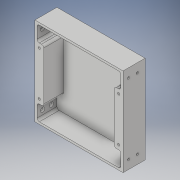
# Autodesk Inventor part: wheel core
Saved by Autodesk Inventor 2018 (Build 220112000, 112)
## iProperties
Created: 2018-08-07
Part Number: wheel core
Material: Generic
Document SubType Name: Modeling
Designer: Cole Tucker
Density: 1 g/cm^3
Appearance: Default
Author: Cole Tucker
Autodesk Inventor part; units mm, degrees
ref_plane "YZ Plane" through (0, 0, 0) normal (1, 0, 0) x (0, 1, 0)
ref_plane "XZ Plane" through (0, 0, 0) normal (0, 1, 0) x (-1, 0, 0)
sketch "Sketch1" plane through (0, 0, 0) normal (0, 0, 1) x (1, 0, 0)
  line L0 (0, 0) -> (127, 0)
  line L1 (127, 0) -> (127, 127)
  line L2 (127, 127) -> (0, 127)
  line L3 (0, 127) -> (0, 0)
  dimension "d0" = 127
  dimension "d1" = 127
  constraints: 8 end point, 2 parallel, 1 horizontal, 1 perpendicular
  measures "d0" distance of L2.end L1.end
  measures "d1" distance of L1.end L0.end
extrude "Extrusion1" add sketch "Sketch1" along normal blind 31.75
shell "Shell1" thickness 3.175 removed faces 1 at (42.3333, 84.6667, 31.75)
sketch "Sketch3" plane through (3.175, 3.175, 3.175) normal (1, 0, 0) x (0, 0, -1)
  line L0 (0, 0) -> (-28.575, 0) construction
  line L1 (-14.2875, 0) -> (-14.2875, 120.65) construction
  line L2 (0, 120.65) -> (-28.575, 120.65) construction
  line L3 (-14.2875, 120.65) -> (-20.6375, 120.65) construction
  line L4 (-20.6375, 120.65) -> (-20.6375, 111.125) construction
  line L5 (-20.6375, 111.125) -> (-14.2875, 111.125) construction
  line L6 (-14.2875, 111.125) -> (-14.2875, 120.65) construction
  line L7 (-14.2875, 120.65) -> (-7.9375, 120.65) construction
  line L8 (-7.9375, 120.65) -> (-7.9375, 111.125) construction
  line L9 (-7.9375, 111.125) -> (-14.2875, 111.125) construction
  line L10 (-14.2875, 111.125) -> (-14.2875, 120.65) construction
  line L11 (-14.2875, 0) -> (-20.6375, 0) construction
  line L12 (-20.6375, 0) -> (-20.6375, 9.525) construction
  line L13 (-20.6375, 9.525) -> (-14.2875, 9.525) construction
  line L14 (-14.2875, 9.525) -> (-14.2875, 0) construction
  line L15 (-14.2875, 0) -> (-7.9375, 0) construction
  line L16 (-7.9375, 0) -> (-7.9375, 9.525) construction
  line L17 (-7.9375, 9.525) -> (-14.2875, 9.525) construction
  line L18 (-14.2875, 9.525) -> (-14.2875, 0) construction
  point P0 (3.175, -3.175)
  dimension "d5" = 6.35
  dimension "d6" = 9.525
  dimension "d7" = 6.35
  dimension "d8" = 6.35
  dimension "d9" = 9.525
  dimension "d10" = 6.35
  dimension "d11" = 9.525
  constraints: 34 end point, 8 parallel, 4 coincident, 4 horizontal, 4 perpendicular, 2 midpoint, 1 point on line
  measures "d5" distance of L5.end L4.end
  measures "d6" distance of L4.end L3.end
  measures "d7" distance of L8.end L9.end
  measures "d8" distance of L12.end L13.end
  measures "d9" distance of L11.end L12.end
  measures "d10" distance of L17.end L16.end
  measures "d11" distance of L16.end L15.end
hole "Hole1" at (3.175, 12.7, 23.8125) at (3.175, 12.7, 11.1125) at (3.175, 114.3, 23.8125) at (3.175, 114.3, 11.1125) direction (-1, 0, 0) diameter 3.175 depth 15.6718 tip angle 118 countersink diameter 6.35 countersink angle 82
ref_plane "Work Plane1" through (63.5, 0, 0) normal (1, 0, 0) x (0, 0, -1)
sketch "Sketch4" plane through (3.175, 3.175, 3.175) normal (0, 0, 1) x (1, 0, 0)
  line L0 (0, 0) -> (0, 120.65) construction
  line L1 (0, 120.65) -> (0, 98.425) construction
  line L2 (0, 0) -> (120.65, 0) construction
  line L3 (0, 0) -> (0, 22.225) construction
  line L4 (0, 98.425) -> (9.525, 98.425)
  line L5 (9.525, 98.425) -> (9.525, 22.225)
  line L6 (9.525, 22.225) -> (0, 22.225)
  line L7 (0, 22.225) -> (0, 98.425)
  point P0 (-3.175, -3.175)
  dimension "d19" = 22.225
  dimension "d20" = 22.225
  dimension "d21" = 9.525
  constraints: 12 end point, 2 parallel, 2 point on line, 1 horizontal, 1 perpendicular
  measures "d19" distance of L0.end L1.end
  measures "d20" distance of L0.start L3.end
  measures "d21" distance of L5.end L6.end
extrude "Extrusion2" add sketch "Sketch4" along normal up to surface (28.575 mm away)
sketch "Sketch5" plane through (0, 0, 31.75) normal (0, 0, 1) x (1, 0, 0)
  line L0 (12.7, 101.6) -> (12.7, 25.4) construction
  line L1 (12.7, 25.4) -> (6.35, 25.4) construction
  line L2 (6.35, 25.4) -> (6.35, 31.75) construction
  line L3 (6.35, 31.75) -> (12.7, 31.75) construction
  line L4 (12.7, 31.75) -> (12.7, 25.4) construction
  line L5 (12.7, 101.6) -> (6.35, 101.6) construction
  line L6 (6.35, 101.6) -> (6.35, 95.25) construction
  line L7 (6.35, 95.25) -> (12.7, 95.25) construction
  line L8 (12.7, 95.25) -> (12.7, 101.6) construction
  point P0 (0, 0)
  dimension "d24" = 6.35
  dimension "d25" = 6.35
  dimension "d26" = 6.35
  dimension "d27" = 6.35
  constraints: 16 end point, 4 parallel, 2 coincident, 2 horizontal, 2 perpendicular
  measures "d24" distance of L2.end L3.end
  measures "d25" distance of L1.end L2.end
  measures "d26" distance of L7.end L6.end
  measures "d27" distance of L6.end L5.end
hole "Hole2" at (6.35, 95.25, 31.75) at (6.35, 31.75, 31.75) direction (0, 0, -1) diameter 3.175 depth 12.7 tip angle 118
mirror "Mirror2" about plane through (63.5, 0, 0) normal (1, 0, 0) of "Hole1", "Extrusion2", "Hole2"
fillet "Fillet1" radius 3.175 12 edges at (3.175, 123.825, 17.4625) (12.7, 101.6, 17.4625) (3.175, 101.6, 17.4625) (12.7, 25.4, 17.4625) (3.175, 25.4, 17.4625) (3.175, 3.175, 17.4625) (123.825, 3.175, 17.4625) (123.825, 25.4, 17.4625) (114.3, 25.4, 17.4625) (114.3, 101.6, 17.4625) (123.825, 101.6, 17.4625) (123.825, 123.825, 17.4625)
body "Solid1"
